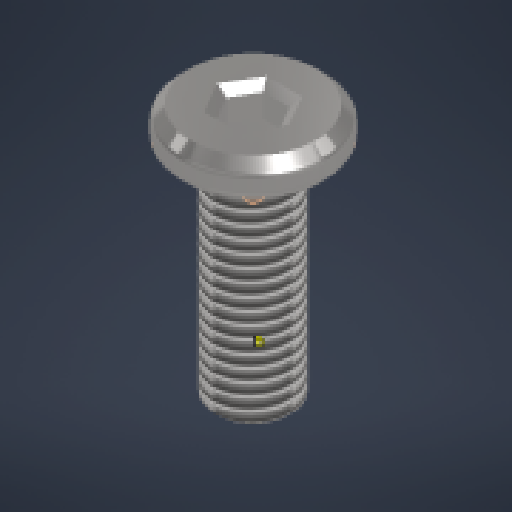
# Autodesk Inventor part: M5-D6-8mm_Screw
Saved by Autodesk Inventor 2024.3 (Build 283343000, 343)
## iProperties
Created: 2025-01-10
Part Number: M5-D6-8mm_Screw
Material: 스테인리스스틸
Document SubType Name: Modeling
Designer: ASUS
Density: 8 g/cm^3
Appearance: 반연마
Author: ASUS
Autodesk Inventor part; units mm, degrees
ref_plane "YZ Plane" through (0, 0, 0) normal (1, 0, 0) x (0, 1, 0)
ref_plane "XZ Plane" through (0, 0, 0) normal (0, 1, 0) x (-1, 0, 0)
ref_plane "XY Plane" through (0, 0, 0) normal (0, 0, 1) x (1, 0, 0)
sketch "스케치1" plane through (0, 0, 0) normal (0, 0, 1) x (1, 0, 0)
  line L0 (0, 0) -> (0, 2.5)
  line L1 (0, 2.5) -> (5.25, 2.5)
  line L2 (5.25, 2.5) -> (5.25, 0)
  line L3 (5.25, 0) -> (0, 0)
  line L4 (0, 2.5) -> (0, 10.5)
  line L5 (0, 10.5) -> (3, 10.5)
  line L6 (3, 10.5) -> (3, 2.5)
  line L7 (3, 2.5) -> (0, 2.5)
  dimension "d0" = 2.5
  dimension "d1" = 5.25
  dimension "d2" = 8
  dimension "d3" = 3
  constraints: 16 end point, 4 parallel, 2 perpendicular, 2 vertical
  measures "d0" distance of L0.start L0.end
  measures "d1" distance of L0.end L1.end
  measures "d2" distance of L0.end L4.end
  measures "d3" distance of L4.end L5.end
revolve "회전1" add sketch "스케치1" angle 360 about axis through (0, 2.5, 0) along (0, 1, 0)
sketch "스케치2" plane through (0, 10.5, 0) normal (0, 1, 0) x (1, 0, 0)
  circle A0 centre (0, 0) radius 3 projected
  circle A1 centre (0, 0) radius 2.5
  dimension "d5" = 5
  constraints: 1 centre point, 1 coincident
  measures "d5" diameter of A1
extrude "돌출1" cut sketch "스케치2" against normal up to surface (8 mm away) contours A1
thread "스레드1" size "M5x0.8" class "6H" standard "ANSI Metric M Profile" full length
chamfer "모따기1" distance 0.5 angle 45 2 edges at (-5.25, 0, 0) (-5.25, 2.5, 0)
sketch "스케치3" plane through (0, 0, 0) normal (0, -1, 0) x (1, 0, 0)
  circle A0 centre (0, 0) radius 2.5 projected
  line L0 (1.7321, 0) -> (0.866, -1.5)
  line L1 (0.866, -1.5) -> (-0.866, -1.5)
  line L2 (-0.866, -1.5) -> (-1.7321, 0)
  line L3 (-1.7321, 0) -> (-0.866, 1.5)
  line L4 (-0.866, 1.5) -> (0.866, 1.5)
  line L5 (0.866, 1.5) -> (1.7321, 0)
  dimension "d13" = 3
  constraints: 12 end point, 1 coincident, 13 other
  measures "d13" distance between parallel lines of L1 L4
extrude "돌출2" cut sketch "스케치3" against normal blind 2 contours L0 L1 L2 L3 L4 L5
chamfer "모따기2" distance 0.5 angle 45 6 edges at (1.299, 0, 0.75) (1.299, 0, -0.75) (0, 0, -1.5) (-1.299, 0, -0.75) (-1.299, 0, 0.75) (0, 0, 1.5)
ref_plane "작업 평면1" through (0, 16.5, 0) normal (0, 1, 0) x (1, 0, 0)
sketch "스케치4" plane through (0, 16.5, 0) normal (0, 1, 0) x (1, 0, 0)
  circle A0 centre (0, 0) radius 4.75 projected
  line L0 (-2.3094, 0) -> (-1.1547, 2) projected
  line L1 (-1.1547, -2) -> (-2.3094, 0) projected
  line L2 (1.1547, -2) -> (-1.1547, -2) projected
  line L3 (2.3094, 0) -> (1.1547, -2) projected
  line L4 (1.1547, 2) -> (2.3094, 0) projected
  line L5 (-1.1547, 2) -> (1.1547, 2) projected
  line L6 (-0.866, -1.5) -> (0.866, -1.5) projected
  line L7 (-1.7321, 0) -> (-0.866, -1.5) projected
  line L8 (-0.866, 1.5) -> (-1.7321, 0) projected
  line L9 (0.866, 1.5) -> (-0.866, 1.5) projected
  line L10 (1.7321, 0) -> (0.866, 1.5) projected
  line L11 (0.866, -1.5) -> (1.7321, 0) projected
extrude "돌출3" add sketch "스케치4" along normal blind 2.3 contours A0 | L0 L5 L4 L3 L2 L1 | L7 L8 L9 L10 L11 L6
sketch "스케치5" plane through (0, 16.5, 0) normal (0, -1, 0) x (1, 0, 0)
  circle A0 centre (0, 0) radius 2.5 projected
  circle A1 centre (0, 0) radius 3 projected
  circle A2 centre (0, 0) radius 2.45
  dimension "d22" = 0.05
  constraints: 1 centre point
  measures "d22" radial gap between concentric circles of A0 A2
extrude "돌출4" add sketch "스케치5" along normal up to surface (14 mm away) contours A2
sketch "스케치6" plane through (0, 18.8, 0) normal (0, 1, 0) x (1, 0, 0)
  line L0 (-0.866, -1.5) -> (0.866, -1.5) projected
  line L1 (-1.7321, 0) -> (-0.866, -1.5) projected
  line L2 (-0.866, 1.5) -> (-1.7321, 0) projected
  line L3 (0.866, 1.5) -> (-0.866, 1.5) projected
  line L4 (1.7321, 0) -> (0.866, 1.5) projected
  line L5 (0.866, -1.5) -> (1.7321, 0) projected
  point P0 (0, 0)
extrude "돌출5" cut sketch "스케치6" against normal blind 2
chamfer "모따기3" distance 0.5 angle 45 7 edges at (-4.75, 16.5, 0) (0, 18.8, 1.5) (-1.299, 18.8, 0.75) (-1.299, 18.8, -0.75) (0, 18.8, -1.5) (1.299, 18.8, -0.75) (1.299, 18.8, 0.75)
chamfer "모따기4" distance 0.7 angle 45 1 edges at (-4.75, 18.8, 0)
fillet "모깎기1" radius 0.5 2 edges at (-4.75, 18.1, 0) (-4.75, 17, 0)
sketch "스케치7" plane through (0, 10.5, 0) normal (0, 1, 0) x (1, 0, 0)
  circle A0 centre (0, 0) radius 2.5 projected
  circle A1 centre (0, 0) radius 3 projected
  circle A2 centre (0, 0) radius 5.25 projected
extrude "돌출6" cut sketch "스케치7" against normal up to surface (10.5 mm away) contours A1 | A2
sketch "스케치8" plane through (0, 0, 0) normal (0, -1, 0) x (1, 0, 0)
  circle A0 centre (0, 0) radius 4.25 projected
  circle A1 centre (0, 0) radius 4.6036 projected
  circle A2 centre (0, 0) radius 2.5 projected
  line L0 (-2.3094, 0) -> (-1.1547, -2) projected
  line L1 (-1.1547, 2) -> (-2.3094, 0) projected
  line L2 (1.1547, 2) -> (-1.1547, 2) projected
  line L3 (2.3094, 0) -> (1.1547, 2) projected
  line L4 (1.1547, -2) -> (2.3094, 0) projected
  line L5 (-1.1547, -2) -> (1.1547, -2) projected
extrude "돌출7" cut sketch "스케치8" against normal up to surface (2.5 mm away) contours A2 | L1 L2 L3 L4 L5 L0
sketch "스케치9" plane through (0, 16.5, 0) normal (0, -1, 0) x (1, 0, 0)
  circle A0 centre (0, 0) radius 2.45 projected
  circle A1 centre (0, 0) radius 4.25 projected
  circle A2 centre (0, 0) radius 2.5
  dimension "d43" = 5
  constraints: 1 centre point, 1 coincident
  measures "d43" diameter of A2
extrude "돌출8" add sketch "스케치9" along normal up to surface (14 mm away) contours A2
chamfer "모따기6" distance 0.25 angle 45 1 edges at (-2.5, 2.5, 0)
thread "스레드3" size "M5x0.8" class "6g" standard "ANSI Metric M Profile" full length
